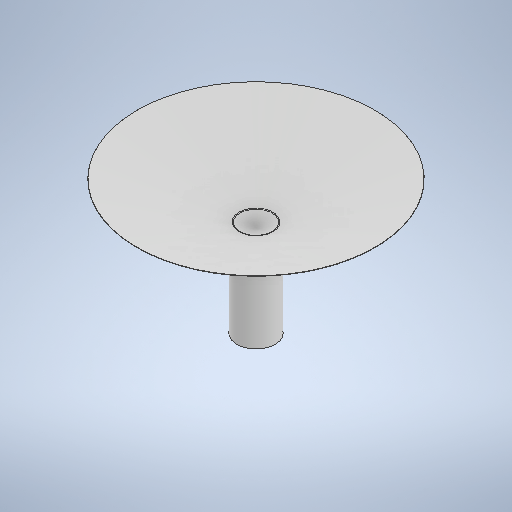
# Autodesk Inventor part: small_membrane
Saved by Autodesk Inventor 2025.2 (Build 292293000, 293)
## iProperties
Created: 2025-03-05
Part Number: small_membrane
Material: Generic
Document SubType Name: Modeling
Designer: fiste
Density: 1 g/cm^3
Appearance: Default
Author: fiste
Autodesk Inventor part; units mm, degrees
ref_plane "YZ Plane" through (0, 0, 0) normal (1, 0, 0) x (0, 1, 0)
ref_plane "XZ Plane" through (0, 0, 0) normal (0, 1, 0) x (-1, 0, 0)
ref_plane "XY Plane" through (0, 0, 0) normal (0, 0, 1) x (1, 0, 0)
sketch "Sketch2" plane through (0, 0, 0) normal (0, 1, 0) x (-1, 0, 0)
  line L0 (37, 0) -> (0, -13.4669)
  line L1 (37, 0) -> (76.3746, 0) construction
  line L2 (0, -13.4669) -> (0, -13.5669)
  line L3 (0, -13.5669) -> (37.0321, -0.0883)
  line L4 (37.0321, -0.0883) -> (37, 0)
  line L5 (0, -16.2803) -> (0, 2.7134) projected
  point P0 (0, 0)
  dimension "d5" = 160
  dimension "d6" = 0.1
  dimension "d7" = 110
  dimension "d8" = 70
  constraints: 10 end point, 1 equal length, 1 horizontal, 1 perpendicular, 1 vertical
  measures "d5" angle of L0 L1
  measures "d6" distance of L0.end L2.end
  measures "d7" angle of L2 L0
  measures "d8" angle of L3 L2
revolve "Revolution2" add sketch "Sketch2" angle 360 about axis through (0, 0, -10) along (0, 0, 1)
sketch "Sketch3" plane through (0, 0, 0) normal (0, 1, 0) x (-1, 0, 0)
  line L0 (-37, 0) -> (0, -13.4669) projected
  line L1 (-5, -11.647) -> (-5, -41.647)
  line L2 (-5, -41.647) -> (-6, -41.647)
  line L3 (-6, -41.647) -> (-6, -11.647)
  line L4 (-6, -11.647) -> (-5, -11.647)
  line L5 (0, -37.9765) -> (0, 6.3294) projected
  point P0 (0, 0)
  dimension "d10" = 30
  dimension "d11" = 1
  dimension "d12" = 90
  dimension "d13" = 30
  dimension "d14" = 90
  constraints: 8 end point, 2 perpendicular, 1 point on line, 1 vertical
  measures "d10" distance of L1.start L1.end
  measures "d11" distance of L1.end L2.end
  measures "d12" angle of L1 L2
  measures "d13" distance of L2.end L3.end
  measures "d14" angle of L2 L3
revolve "Revolution3" add sketch "Sketch3" angle 360 about axis through (0, 0, -10) along (0, 0, 1)
body "Solid2"
